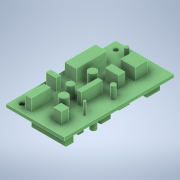
# Autodesk Inventor part: printplaat
Saved by Autodesk Inventor 2022 (Build 260153000, 153)
## iProperties
Created: 2022-02-24
Part Number: printplaat
Material: Generic
Document SubType Name: Modeling
Designer: woutr
Density: 1 g/cm^3
Appearance: Smooth - Dark Forest Green
Author: woutr
Autodesk Inventor part; units mm, degrees
ref_plane "YZ Plane" through (0, 0, 0) normal (1, 0, 0) x (0, 1, 0)
ref_plane "XZ Plane" through (0, 0, 0) normal (0, 1, 0) x (-1, 0, 0)
ref_plane "XY Plane" through (0, 0, 0) normal (0, 0, 1) x (1, 0, 0)
sketch "Sketch1" plane through (0, 0, 0) normal (0, 1, 0) x (-1, 0, 0)
  line L0 (0, 0) -> (37, 0)
  line L1 (37, 0) -> (37, -70)
  line L2 (37, -70) -> (0, -70)
  line L3 (0, -70) -> (0, 0)
  dimension "d0" = 37
  dimension "d1" = 70
  constraints: 8 end point, 2 parallel, 1 horizontal, 1 perpendicular
  measures "d0" distance of L1.end L2.end
  measures "d1" distance of L0.end L1.end
extrude "Extrusion1" add sketch "Sketch1" along normal blind 2
sketch "Sketch2" plane through (0, 2, 0) normal (0, 1, 0) x (1, 0, 0)
  circle A0 centre (-32, 5) radius 1.5
  circle A1 centre (-32, 65) radius 1.5
  line L0 (-37, 70) -> (-37, 0) projected
  line L1 (-37, 0) -> (0, 0) projected
  line L2 (0, 70) -> (-37, 70) projected
  dimension "d4" = 3
  dimension "d5" = 3
  dimension "d6" = 5
  dimension "d11" = 60
  dimension "d12" = 5
  constraints: 2 centre point, 1 vertical alignment
  measures "d4" diameter of A0
  measures "d5" diameter of A1
  measures "d6" distance from line of L0 A0.centre
  measures "d11" distance of A1.centre A0.centre
  measures "d12" distance from line of L1 A0.centre
extrude "Extrusion2" cut sketch "Sketch2" against normal through all
sketch "Sketch3" plane through (0, 2, 0) normal (0, 1, 0) x (1, 0, 0)
  line L0 (-8.0701, 61.2061) -> (-17.4041, 61.2061)
  line L1 (-17.4041, 61.2061) -> (-17.4041, 53.4277)
  line L2 (-17.4041, 53.4277) -> (-8.0701, 53.4277)
  line L3 (-8.0701, 53.4277) -> (-8.0701, 61.2061)
  line L4 (-26.252, 53.4277) -> (-33.447, 53.4277)
  line L5 (-33.447, 53.4277) -> (-33.447, 33.8845)
  line L6 (-33.447, 33.8845) -> (-26.252, 33.8845)
  line L7 (-26.252, 33.8845) -> (-26.252, 53.4277)
  line L8 (-14.1955, 35.8291) -> (-11.4731, 35.8291)
  line L9 (-11.4731, 35.8291) -> (-11.4731, 22.3142)
  line L10 (-11.4731, 22.3142) -> (-14.1955, 22.3142)
  line L11 (-14.1955, 22.3142) -> (-14.1955, 35.8291)
  line L12 (-8.9451, 47.8856) -> (-17.4041, 47.8856)
  line L13 (-17.4041, 47.8856) -> (-17.4041, 43.6561)
  line L14 (-17.4041, 43.6561) -> (-8.9451, 43.6561)
  line L15 (-8.9451, 43.6561) -> (-8.9451, 47.8856)
  line L16 (-7.0978, 10.1605) -> (-12.0565, 10.1605)
  line L17 (-12.0565, 10.1605) -> (-12.0565, 5.299)
  line L18 (-12.0565, 5.299) -> (-7.0978, 5.299)
  line L19 (-7.0978, 5.299) -> (-7.0978, 10.1605)
  line L20 (-24.113, 3.0627) -> (-28.0994, 3.0627)
  line L21 (-28.0994, 3.0627) -> (-28.0994, 15.3137)
  line L22 (-28.0994, 15.3137) -> (-24.113, 15.3137)
  line L23 (-24.113, 15.3137) -> (-24.113, 3.0627)
  line L24 (-27.516, 22.3142) -> (-33.9332, 22.3142)
  line L25 (-33.9332, 22.3142) -> (-33.9332, 25.2311)
  line L26 (-33.9332, 25.2311) -> (-27.516, 25.2311)
  line L27 (-27.516, 25.2311) -> (-27.516, 22.3142)
  circle A0 centre (-19.8349, 37.871) radius 2.5092
  circle A1 centre (-19.8349, 23.7727) radius 2.1324
  circle A2 centre (-5.7366, 37.1904) radius 1.481
  circle A3 centre (-5.7366, 18.8139) radius 0.7011
  circle A4 centre (-15.5567, 15.3137) radius 2.6288
  circle A5 centre (-22.3441, 62.1784) radius 1.2864
  point P0 (0, 0)
  constraints: 56 end point, 14 parallel, 7 horizontal, 7 perpendicular, 6 centre point, 3 point on line
extrude "Extrusion3" add sketch "Sketch3" along normal blind 8
sketch "Sketch4" plane through (0, 0, 0) normal (0, -1, 0) x (1, 0, 0)
  line L0 (-18.8626, -58.0947) -> (-15.5567, -58.0947)
  line L1 (-15.5567, -58.0947) -> (-15.5567, -54.2055)
  line L2 (-15.5567, -54.2055) -> (-18.8626, -54.2055)
  line L3 (-18.8626, -54.2055) -> (-18.8626, -58.0947)
  line L4 (-18.3764, -25.9117) -> (-11.4731, -25.9117)
  line L5 (-11.4731, -25.9117) -> (-11.4731, -21.7308)
  line L6 (-11.4731, -21.7308) -> (-18.3764, -21.7308)
  line L7 (-18.3764, -21.7308) -> (-18.3764, -25.9117)
  line L8 (-6.4172, -48.1773) -> (-11.4731, -48.1773)
  line L9 (-11.4731, -48.1773) -> (-11.4731, -41.274)
  line L10 (-11.4731, -41.274) -> (-6.4172, -41.274)
  line L11 (-6.4172, -41.274) -> (-6.4172, -48.1773)
  line L12 (-32.0858, -34.1762) -> (-17.2097, -34.1762)
  line L13 (-17.2097, -34.1762) -> (-17.2097, -43.0241)
  line L14 (-17.2097, -43.0241) -> (-32.0858, -43.0241)
  line L15 (-32.0858, -43.0241) -> (-32.0858, -34.1762)
  line L16 (-33.1553, -59.9421) -> (-23.0434, -59.9421)
  line L17 (-23.0434, -59.9421) -> (-23.0434, -48.1773)
  line L18 (-23.0434, -48.1773) -> (-33.1553, -48.1773)
  line L19 (-33.1553, -48.1773) -> (-33.1553, -59.9421)
  line L20 (-32.0858, -25.9117) -> (-22.0711, -25.9117)
  line L21 (-22.0711, -25.9117) -> (-22.0711, -14.1469)
  line L22 (-22.0711, -14.1469) -> (-32.0858, -14.1469)
  line L23 (-32.0858, -14.1469) -> (-32.0858, -25.9117)
  line L24 (-25.1825, -4.3267) -> (-3.2086, -4.3267)
  line L25 (-3.2086, -4.3267) -> (-3.2086, -9.091)
  line L26 (-3.2086, -9.091) -> (-25.1825, -9.091)
  line L27 (-25.1825, -9.091) -> (-25.1825, -4.3267)
  circle A0 centre (-5.7366, -18.8139) radius 0.7011 projected
  line L28 (-13.2232, -14.8275) -> (-5.7366, -14.8275)
  line L29 (-5.7366, -14.8275) -> (-5.7366, -18.1128)
  line L30 (-5.7366, -18.1128) -> (-13.2232, -18.1128)
  line L31 (-13.2232, -18.1128) -> (-13.2232, -14.8275)
  line L32 (-7.6811, -34.1762) -> (-4.4726, -34.1762)
  line L33 (-4.4726, -34.1762) -> (-4.4726, -27.9535)
  line L34 (-4.4726, -27.9535) -> (-7.6811, -27.9535)
  line L35 (-7.6811, -27.9535) -> (-7.6811, -34.1762)
  line L36 (-10.6953, -65.6787) -> (-4.4726, -65.6787)
  line L37 (-4.4726, -65.6787) -> (-4.4726, -57.3169)
  line L38 (-4.4726, -57.3169) -> (-10.6953, -57.3169)
  line L39 (-10.6953, -57.3169) -> (-10.6953, -65.6787)
  circle A1 centre (-17.6958, -65.6787) radius 2.4366
  circle A2 centre (-16.7235, -48.1773) radius 2.7842
  circle A3 centre (-11.4731, -33.4956) radius 1.7008
  circle A4 centre (-28.0994, -30.3843) radius 1.1308
  circle A5 centre (-17.6958, -15.5081) radius 3.5421
  circle A6 centre (-4.4726, -23.092) radius 1.8576
  point P0 (0, 0)
  constraints: 80 end point, 20 parallel, 10 horizontal, 10 perpendicular, 6 centre point, 4 point on line, 1 vertical alignment, 1 other
extrude "Extrusion4" add sketch "Sketch4" along normal blind 7 contours L3 L2 L1 L0 | L7 L6 L5 L4 | L8 L9 L10 L11 | L12 L13 L14 L15 | L19 L18 L17 L16 | L23 L22 L21 L20 | L24 L25 L26 L27 | L30 L31 L28 L29 | L35 L34 L33 L32 | L39 L38 L37 L36 | A1 | A2 | A3 | A4 | A5 | A6
body "Solid1"
